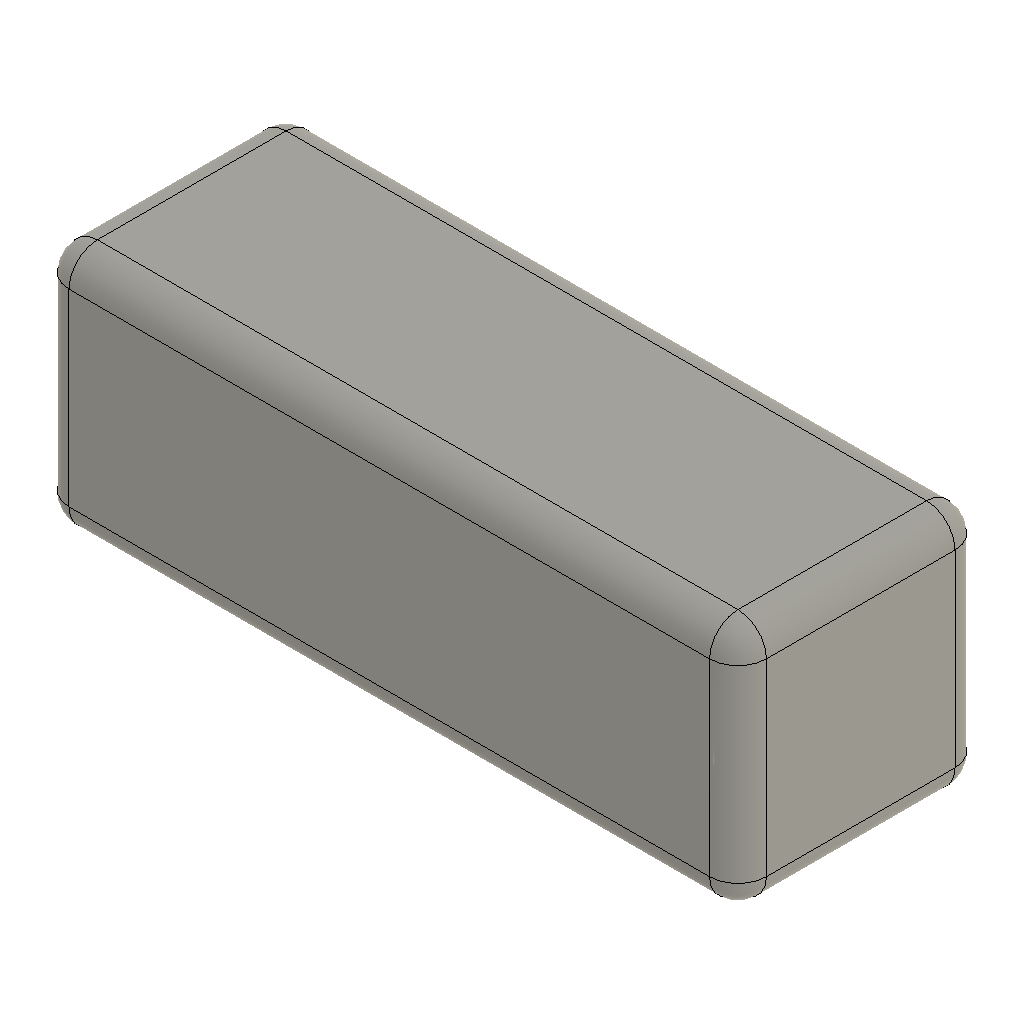
Connector (Autodesk Fusion 360 design; units mm, degrees)
Autodesk Fusion 360 part; units mm, degrees
sketch "Sketch1" plane through (0, 0, 0) normal (1, 0, 0) x (0, 1, 0)
  line L0 (1.725, -1.725) -> (-1.725, -1.725)
  line L1 (-1.725, -1.725) -> (-1.725, 1.725)
  line L2 (-1.725, 1.725) -> (1.725, 1.725)
  line L3 (1.725, 1.725) -> (1.725, -1.725)
  line L4 (1.725, -1.725) -> (-1.725, 1.725) construction
  line L5 (-1.725, -1.725) -> (1.725, 1.725) construction
  dimension "d10" = 3.45
  dimension "d11" = 3.45
  constraint horizontal L0
  constraint perpendicular L0 L1
  constraint parallel L0 L2
  constraint parallel L1 L3
  constraint coincident L4 origin
  constraint coincident L5 origin
  measures "d10" distance of L1.end L2.end
  measures "d11" distance of L0.end L1.end
extrude "Extrude1" add sketch "Sketch1" along normal blind 4.9
extrude "Extrude2" add 1 faces at (0, -0.575, 0.575) along direction (-1, 0, 0) blind 4.9
fillet "Fillet1" radius 0.4 6 faces at (4.9, -0.575, 0.575) (-4.9, -0.575, 0.575) (1.6333, -0.575, 1.725) (1.6333, -1.725, -0.575) (1.6333, 1.725, 0.575) (1.6333, 0.575, -1.725)
equation "d11 = d10"
named bodies: "Connector"
